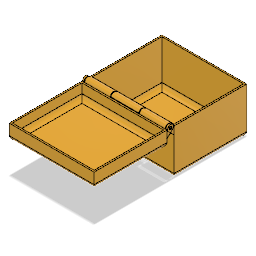
New_HingedBox70mm_v1 (Autodesk Fusion 360 design; units mm, degrees)
Autodesk Fusion 360 part; units mm, degrees
note: some values were not read from the file. Chosen so that the rebuilt part matches the saved one: which bodies a step acts on; which face or edge a step refers to. Set by a fixed rule: which sketch regions a step uses.
sketch "Box" plane through (0, 0, 0) normal (0, 1, 0) x (1, 0, 0) in component "Bottom"
  line L0 (0, 0) -> (-70, 0)
  line L1 (-70, 0) -> (-70, 60)
  line L2 (-70, 60) -> (0, 60)
  line L3 (0, 60) -> (0, 0)
  dimension "d1" = 70
  dimension "d2" = 60
extrude "Extrude1" add sketch "Box" along normal blind 50 makes body 1 in component "Bottom"
shell "Shell1" thickness 1.3 removed faces 0 bodies 1 in component "Bottom"
ref_plane "WorkPlane1" through (-35, 37.5, -30) normal (0, 1, 0) x (0, 0, 1) in component "Bottom"
split "Split1" by plane through (-35, 37.5, -30) normal (0, 1, 0) bodies 1 makes body 2 at (-23.3333, 50, -20) in component "Bottom"
sketch "Hinge" plane through (0, 0, 0) normal (1, 0, 0) x (0, 0, -1) in component "Bottom"
  line L0 (60, 37.5) -> (0, 37.5)
  line L1 (0, 37.5) -> (0, 0)
  line L2 (0, 0) -> (60, 0)
  line L3 (60, 0) -> (60, 37.5)
  line L4 (0, 37.5) -> (-2.95, 37.5)
  circle A0 centre (-2.95, 37.5) radius 2.45
  circle A1 centre (-2.95, 37.5) radius 1.15
  circle A2 centre (-2.95, 37.5) radius 0.65
  line L5 (0, 31.0852) -> (-4.6824, 35.7676)
  line L6 (0, 37.5) -> (0, 50)
  line L7 (0, 43.9148) -> (-4.6824, 39.2324)
  dimension "d10" = 2.95
  dimension "d11" = 1.3
  dimension "d12" = 0.5
  dimension "d13" = 1.3
  dimension "d14" = 45
  dimension "d15" = 45
  measures "d10" distance of L1.end
  measures "d11" diameter of A2
  measures "d12" distance of A1 A2
  measures "d13" distance of A0 A1
  measures "d14" angle of L1 L5
  measures "d15" angle of L6 L7
extrude "Extrude2" add sketch "Hinge" against normal up to surface (70 mm away) separate body contours L1 L4 A0 L5 | A0 makes body 3 in component "Bottom"
extrude "Extrude3" add sketch "Hinge" against normal up to surface (70 mm away) separate body contours L4 A0 L6 L7 | A0 | A1 | A2 makes body 4 in component "Bottom"
extrude "Extrude4" add sketch "Hinge" against normal up to surface (70 mm away) separate body contours A1 makes body 5 in component "Bottom"
sketch "Sketch3" plane through (0, 37.5, 0) normal (0, 1, 0) x (-1, 0, 0) in component "Bottom"
  line L0 (0, 0) -> (0, -60)
  line L1 (0, -60) -> (70, -60)
  line L2 (70, -60) -> (70, 0)
  line L3 (70, 0) -> (0, 0)
  line L4 (1.3, -58.7) -> (1.3, -1.3)
  line L5 (1.3, -1.3) -> (68.7, -1.3)
  line L6 (68.7, -1.3) -> (68.7, -58.7)
  line L7 (68.7, -58.7) -> (1.3, -58.7)
  line L8 (0, 0) -> (1.3, 0)
  line L9 (1.3, 0) -> (1.3, 5.5)
  line L10 (1.3, 5.5) -> (0, 5.5)
  line L11 (0, 5.5) -> (0, 0)
  line L12 (1.3, 0) -> (1.8, 0)
  line L13 (1.8, 0) -> (1.8, 5.5)
  line L14 (1.8, 5.5) -> (1.3, 5.5)
  line L15 (1.3, 5.5) -> (1.3, 0)
  line L16 (35, 0) -> (35, 10) construction
  line L17 (35, 0) -> (23.5, 0) construction
  line L18 (23.5, 0) -> (23, 0)
  line L19 (23, 0) -> (23, 5.5)
  line L20 (23, 5.5) -> (23.5, 5.5)
  line L21 (23.5, 5.5) -> (23.5, 0)
  line L22 (47, 5.5) -> (46.5, 5.5)
  line L23 (68.7, 0) -> (68.2, 0)
  line L24 (68.2, 5.5) -> (68.7, 5.5)
  line L25 (46.5, 0) -> (47, 0)
  line L26 (68.7, 0) -> (68.7, 5.5)
  line L27 (68.2, 0) -> (68.2, 5.5)
  line L28 (47, 0) -> (47, 5.5)
  line L29 (46.5, 5.5) -> (46.5, 0)
  line L30 (70, 0) -> (68.7, 0)
  line L31 (70, 5.5) -> (70, 0)
  line L32 (68.7, 5.5) -> (70, 5.5)
  line L33 (35, 0) -> (46.5, 0) construction
  dimension "d22" = 5.5
  dimension "d23" = 1.3
  dimension "d24" = 0.5
  dimension "d25" = 5.5
  dimension "d26" = 11.5
  dimension "d27" = 5.5
  dimension "d28" = 0.5
  measures "d22" distance of L0.start
  measures "d27" distance of L0.start
extrude "Extrude5" cut sketch "Sketch3" along normal through all and the other way through all contours L3 L9 L12 L13 L14 L15 | L3 L18 L19 L20 L21 | L3 L23 L24 L26 L27 | L3 L22 L25 L28 L29 | L4 L5 L6 L7 bodies 3 4 makes body 10 at (-61.1333, 35.7017, 1.2861) makes body 11 at (-1.3, 40.2157, 1.7275) makes body 12 at (-38.8333, 35.7845, 1.2009) makes body 13 at (-68.7, 40.2157, 1.7275) makes body 6 at (-61.1333, 38.4266, 0.682) makes body 7 at (-1.3, 35.062, 0.7443) makes body 8 at (-15.9333, 38.4266, 0.682) makes body 9 at (-68.7, 35.062, 0.7443) in component "Bottom"
delete_body "RemoveBody1" bodies 3 in component "Bottom"
delete_body "RemoveBody2" bodies 4 in component "Bottom"
delete_body "RemoveBody3" bodies 10 in component "Bottom"
copy_body "Body->Comp1" bodies 2 removing the originals makes body 14 in component "Lid"
copy_body "CutPasteBodies1" bodies 5 11 12 13 removing the originals makes body 15 makes body 16 makes body 17 makes body 18 in component "Lid"
fillet "Fillet1" radius 3.5 8 edges at (-35, 50, -60) (0, 50, -30) (-35, 50, 0) (-70, 50, -30) (-35, 48.7, -1.3) (-35, 48.7, -58.7) (-1.3, 48.7, -30) (-68.7, 48.7, -30) on bodies 14 in component "Lid"
fillet "Fillet1'" radius 3.5 8 edges at (0, 0, -30) (-35, 0, -60) (-35, 1.3, -58.7) (-1.3, 1.3, -30) (-68.7, 1.3, -30) (-35, 1.3, -1.3) (-35, 0, 0) (-70, 0, -30) on bodies 1 in component "Bottom"
component "Bottom" placed x (1, 0, 0) y (0, 1, 0) z (0, 0, 1) at (0, 0, 0)
component "Lid" placed x (1, 0, 0) y (0, 1, 0) z (0, 0, 1) at (0, 0, 0)
equation "WallThickness = 1.3 mm" comment "FDM 3DPrinter Thickness"
equation "BoxHeight = 50 mm"
equation "HingeGap = 0.5 mm"
equation "d6 = BoxHeight"
equation "d8 = WallThickness"
equation "d9 = -BoxHeight / 4"
equation "d11 = WallThickness"
equation "d12 = HingeGap"
equation "d13 = WallThickness"
equation "d23 = WallThickness"
equation "d24 = HingeGap"
equation "d28 = HingeGap"
equation "d35 = FilletRadius"
equation "FilletRadius = 3.5 mm"
equation "d37 = FilletRadius"
named bodies: "Bottom", "Lid", "BottomHinge", "TopHinge", "Pin", "BottomHinge (1)", "BottomHinge (2)", "BottomHinge (3)", "BottomHinge (4)", "TopHinge (1)", "TopHinge (2)", "TopHinge (3)", "TopHinge (4)"
